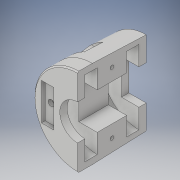
# Autodesk Inventor part: cameraHolder
Saved by Autodesk Inventor 2019.3 (Build 233278000, 278)
## iProperties
Created: 2019-10-29
Part Number: cameraHolder
Material: Generic
Document SubType Name: Modeling
Designer: Ayaz
Density: 1 g/cm^3
Appearance: Default
Mass: 59.2053 g
Surface Area: 200.736 cm^2
Volume: 59.2053 cm^3
Author: Ayaz
Autodesk Inventor part; units mm, degrees
ref_plane "YZ Plane" through (0, 0, 0) normal (1, 0, 0) x (0, 1, 0)
sketch "Sketch1" plane through (0, 0, 0) normal (0, 1, 0) x (-1, 0, 0)
  line L0 (0, 0) -> (0, 35.75)
  line L1 (0, 0) -> (-56, 0)
  line L2 (-56, 0) -> (-56, 33.9625)
  line L3 (11.2, 0) -> (-67.2, 0) projected
  line L4 (-50, 30.1718) -> (-50, 6)
  line L5 (-6, 6) -> (-6, 30.7506)
  line L6 (-6, 30.7506) -> (-50, 30.1718)
  line L7 (-28, 0) -> (-28, 30.4612)
  line L8 (-16, 0) -> (-16, 30.619)
  line L9 (-40, 0) -> (-40, 30.3033)
  line L10 (-50, 6) -> (-40, 6)
  line L11 (-16, 6) -> (-6, 6)
  line L12 (0, 35.75) -> (-12, 35.75)
  line L13 (-12, 35.75) -> (-56, 33.9625)
  dimension "d1" = 33.9625
  dimension "d8" = 35.75
  dimension "d10" = 56
  dimension "d22" = 28
  dimension "d23" = 12
  dimension "d24" = 12
  dimension "d29" = 12
  constraints: 26 end point, 4 point on line, 2 midpoint, 2 parallel, 2 vertical, 1 horizontal, 1 perpendicular
  measures "d1" distance of L1.end L2.end
  measures "d8" distance of L0.start L0.end
  measures "d10" distance of L0.start L1.end
  measures "d22" distance between parallel lines of L0 L7
  measures "d23" distance between parallel lines of L7 L8
  measures "d24" distance between parallel lines of L7 L9
  measures "d29" distance of L0.end L12.end
revolve "Revolution1" add sketch "Sketch1" angle 180 about axis through (-10, 0, 0) along (-1, 0, 0) contours L1 L8 L11 L5 L6 L4 L10 L9 L2 L13 L12 L0 | L1 L7 L6 L8 | L1 L9 L6 L7
ref_plane "Work Plane1" through (6, 0, 0) normal (-1, 0, 0) x (0, 0, -1)
sketch "Sketch3" plane through (6, 0, 0) normal (-1, 0, 0) x (0, 0, -1)
  line L0 (-15, 15) -> (15, 15)
  line L1 (15, 15) -> (15, -15)
  line L2 (15, -15) -> (-15, -15)
  line L3 (-15, -15) -> (-15, 15)
  line L4 (-15, 15) -> (15, -15) construction
  line L5 (15, 15) -> (-15, -15) construction
  point P0 (0, 0)
  dimension "d12" = 30
  dimension "d13" = 30
  constraints: 12 end point, 2 midpoint, 2 parallel, 1 horizontal, 1 perpendicular
  measures "d12" distance of L1.end L2.end
  measures "d13" distance of L0.end L1.end
extrude "Extrusion2" cut sketch "Sketch3" against normal blind 44
sketch "Sketch4" plane through (0, 0, 0) normal (-1, 0, 0) x (0, 0, -1)
  circle A0 centre (0, 0) radius 14.5
  point P0 (0, 0)
  dimension "d16" = 29
  constraints: 1 centre point, 1 coincident
  measures "d16" diameter of A0
extrude "Extrusion3" cut sketch "Sketch4" against normal blind 6
sketch "Sketch5" plane through (56, 0, 0) normal (1, 0, 0) x (0, 0, -1)
  line L0 (14.25, -14.25) -> (-14.25, -14.25)
  line L1 (-14.25, -14.25) -> (-14.25, 14.25)
  line L2 (-14.25, 14.25) -> (14.25, 14.25)
  line L3 (14.25, 14.25) -> (14.25, -14.25)
  line L4 (14.25, -14.25) -> (-14.25, 14.25) construction
  line L5 (-14.25, -14.25) -> (14.25, 14.25) construction
  point P0 (0, 0)
  dimension "d25" = 28.5
  dimension "d26" = 28.5
  constraints: 12 end point, 2 midpoint, 2 parallel, 1 horizontal, 1 perpendicular
  measures "d25" distance of L1.end L2.end
  measures "d26" distance of L0.end L1.end
extrude "Extrusion4" cut sketch "Sketch5" against normal blind 6
chamfer "Chamfer3" distance 1 angle 45 1 edges at (0, 35.75, 0)
sketch "Sketch6" plane through (16, 0, 15) normal (0, -1, 0) x (1, 0, 0)
  line L0 (-16, 19.75) -> (-15, 20.75) projected
  line L1 (-16, -0.5) -> (-16, 19.75) projected
  line L2 (-16, -0.5) -> (-10, -0.5) projected
  line L3 (-10, -0.5) -> (-10, 15.7506) projected
  line L4 (-10, 15.7506) -> (0, 15.619) projected
  line L5 (0, 15.619) -> (0, 0) projected
  line L6 (0, 0) -> (24, 0) projected
  line L7 (24, 0) -> (24, 15.3033) projected
  line L8 (24, 15.3033) -> (34, 15.1718) projected
  line L9 (34, 15.1718) -> (34, -0.75) projected
  line L10 (34, -0.75) -> (40, -0.75) projected
  line L11 (40, 18.9625) -> (40, -0.75) projected
  line L12 (-4, 20.75) -> (40, 18.9625) projected
  line L13 (-15, 20.75) -> (-4, 20.75) projected
  line L14 (-16, -15) -> (40, -15)
  line L15 (40, -0.75) -> (40, -29.25) projected
  line L16 (13, -15) -> (38, -15) construction
  line L17 (12, -15) -> (12, 10)
  line L18 (12, -15) -> (37, -15) construction
  circle A0 centre (12, 10) radius 1.5
  dimension "d46" = 25
  dimension "d47" = 90
  dimension "d48" = 3
  constraints: 8 end point, 2 horizontal, 2 midpoint, 1 centre point, 1 coincident, 1 perpendicular
  measures "d46" distance of L17.start L17.end
  measures "d47" angle of L18 L17
  measures "d48" diameter of A0
extrude "Extrusion5" cut sketch "Sketch6" against normal through all contours A0
ref_plane "Work Plane2" through (0, 15, 0) normal (0, 1, 0) x (-1, 0, 0)
sketch "Sketch7" plane through (0, 15, 0) normal (0, 1, 0) x (-1, 0, 0)
  circle A0 centre (-28, 25) radius 1.5 projected
  arc A1 (-35.5, 25) -> (-20.5, 25) centre (-28, 25) ccw
  spline S0 degree 5 poles (-29.5, 25) (-29.5, 25.2111) (-29.4629, 25.4204) (-29.3897, 25.6231) (-29.2804, 25.8128) (-29.0332, 26.0983) (-28.9152, 26.2048) (-28.7791, 26.2979) (-28.6269, 26.3735) (-28.3307, 26.4697) (-28.1905, 26.4982) (-28.0469, 26.5095) (-27.9041, 26.5034) (-27.5429, 26.4465) (-27.3324, 26.3699) (-27.1499, 26.2607) (-26.9942, 26.1299) (-26.7049, 25.7958) (-26.5873, 25.5835) (-26.513, 25.3527) (-26.4842, 25.1114) (-26.5242, 24.6611) (-26.578, 24.4533) (-26.6719, 24.2502) (-26.8064, 24.0618) (-27.1556, 23.7366) (-27.3724, 23.6017) (-27.6224, 23.5132) (-27.8827, 23.4833) (-28.3338, 23.524) (-28.5277, 23.5752) (-28.7076, 23.6563) (-28.8674, 23.7623) (-29.2025, 24.0647) (-29.3531, 24.2808) (-29.4523, 24.5167) (-29.5, 24.7592) (-29.5, 25) knots 0 0 0 0 0 0 0.12181 0.12181 0.12181 0.12181 0.205743 0.205743 0.205743 0.205743 0.273981 0.273981 0.273981 0.273981 0.384852 0.384852 0.384852 0.384852 0.524069 0.524069 0.524069 0.524069 0.641928 0.641928 0.641928 0.641928 0.764397 0.764397 0.764397 0.764397 0.86105 0.86105 0.86105 0.86105 1 1 1 1 1 1 projected
  line L0 (-12, 35.75) -> (-56, 33.9625) projected
  line L1 (-56, 33.9625) -> (-56, -33.9625) projected
  line L2 (-12, -35.75) -> (-56, -33.9625) projected
  line L3 (-12, 35.75) -> (-12, -35.75) projected
  line L4 (-20.5, 25) -> (-20.5, 35.4047)
  line L5 (-35.5, 25) -> (-35.5, 34.7953)
  point P0 (0, 0)
  dimension "d50" = 15
  constraints: 4 end point, 2 point on circle, 2 point on line, 2 vertical, 1 centre point, 1 coincident, 1 tangent, 1 other
  measures "d50" diameter of A1
extrude "Extrusion7" cut sketch "Sketch7" along normal blind 40 contours L5 L0 L4 A1
sketch "Sketch8" plane through (0, 0, 0) normal (-1, 0, 0) x (0, 0, 1)
  line L0 (0, 0) -> (0, 19.5)
  line L1 (0, 19.5) -> (15, 19.5)
  line L2 (15, 19.5) -> (15, 29.5)
  line L3 (15, 29.5) -> (-15, 29.5)
  line L4 (-15, 29.5) -> (-15, 19.5)
  line L5 (-15, 19.5) -> (0, 19.5)
  dimension "d61" = 19.5
  dimension "d62" = 15
  dimension "d63" = 10
  dimension "d64" = 30
  dimension "d65" = 90
  dimension "d66" = 10
  constraints: 12 end point, 2 perpendicular, 1 horizontal, 1 point on line, 1 vertical
  measures "d61" distance of L0.start L0.end
  measures "d62" distance of L0.end L1.end
  measures "d63" distance of L1.end L2.end
  measures "d64" distance of L2.end L3.end
  measures "d65" angle of L3 L2
  measures "d66" distance of L3.end L4.end
extrude "Extrusion8" cut sketch "Sketch8" against normal blind 3
mirror "Mirror3" about plane through (0, 0, 0) normal (0, 0, 1) of "Extrusion5", "Extrusion7"
sketch "Sketch10" plane through (3, 0, 0) normal (-1, 0, 0) x (0, 0, 1)
  line L0 (15, 19.5) -> (-15, 19.5) projected
  line L1 (15, 29.5) -> (15, 19.5) projected
  line L2 (-15, 29.5) -> (15, 29.5) projected
  line L3 (-15, 19.5) -> (-15, 29.5) projected
  line L4 (-15, 19.5) -> (-15, 29.5) projected
  line L5 (-15, 19.5) -> (15, 29.5)
  circle A0 centre (0, 24.5) radius 2.5
  point P0 (0, 0)
  dimension "d67" = 5
  constraints: 2 end point, 1 centre point, 1 midpoint
  measures "d67" diameter of A0
extrude "Extrusion9" cut sketch "Sketch10" against normal up to next contours A0 L5 | L5 A0
equation "\"d8\" = 0.5 * pipeID"
equation "\"d22\" = 0.5 * d10"
equation "\"d23\" = 2 * wallTh"
equation "\"d24\" = 2 * wallTh"
equation "\"d29\" = 2 * wallTh"
equation "\"d17\" = wallTh"
equation "\"d27\" = wallTh"
equation "\"pipeID\" = 71.5"
equation "\"wallTh\" = 6"
equation "\"taper\" = 0.95"
equation "\"d11\" = -wallTh"
body "Solid1"
